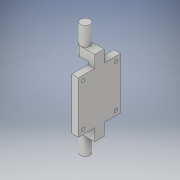
# Autodesk Inventor part: Paltte klein 2.0
Saved by Autodesk Inventor 2018.3 (Build 223284000, 284)
## iProperties
Created: 2018-11-08
Part Number: Paltte klein 2.0
Material: Generisch
Document SubType Name: Modeling
Designer: pgmadmin
Density: 1 g/cm^3
Appearance: Vorgabe
Author: pgmadmin
Autodesk Inventor part; units mm, degrees
ref_plane "YZ Plane" through (0, 0, 0) normal (1, 0, 0) x (0, 1, 0)
ref_plane "XZ Plane" through (0, 0, 0) normal (0, 1, 0) x (-1, 0, 0)
ref_plane "XY Plane" through (0, 0, 0) normal (0, 0, 1) x (1, 0, 0)
sketch "Skizze1" plane through (0, 0, 0) normal (1, 0, 0) x (0, 1, 0)
  line L0 (52.9121, 68.8462) -> (7.9121, 68.8462)
  line L1 (7.9121, 68.8462) -> (7.9121, 13.8462)
  line L2 (7.9121, 13.8462) -> (52.9121, 13.8462)
  line L3 (52.9121, 13.8462) -> (52.9121, 68.8462)
  circle A0 centre (12.9121, 18.8462) radius 1.75
  circle A1 centre (12.9121, 63.8462) radius 1.75
  circle A2 centre (47.9121, 63.8462) radius 1.75
  circle A3 centre (47.9121, 18.8462) radius 1.75
  point P0 (0, 0)
  dimension "d0" = 45
  dimension "d1" = 55
  dimension "d2" = 3.5
  dimension "d3" = 5
  dimension "d4" = 5
  dimension "d5" = 3.5
  dimension "d6" = 5
  dimension "d7" = 3.5
  dimension "d8" = 5
  dimension "d11" = 3.5
  constraints: 8 end point, 4 centre point, 4 coincident, 2 parallel, 1 horizontal, 1 perpendicular
  measures "d0" distance of L1.end L2.end
  measures "d1" distance of L0.end L1.end
  measures "d2" diameter of A0
  measures "d3" distance from line of L1 A0.centre
  measures "d4" distance from line of L2 A0.centre
  measures "d5" diameter of A1
  measures "d6" distance from line of L0 A1.centre
  measures "d7" diameter of A2
  measures "d8" distance from line of L3 A2.centre
  measures "d11" diameter of A3
extrude "Extrusion1" add sketch "Skizze1" along normal blind 7
sketch "Skizze2" plane through (0, 7.9121, 68.8462) normal (0, 0, 1) x (1, 0, 0)
  line L0 (0, 45) -> (0, 0) projected
  line L1 (7, 45) -> (7, 0) projected
  line L2 (0, 17.5) -> (7, 17.5)
  line L3 (7, 17.5) -> (7, 27.5)
  line L4 (7, 27.5) -> (0, 27.5)
  line L5 (0, 27.5) -> (0, 17.5)
  line L6 (0, 45) -> (7, 45) projected
  point P0 (0, -7.9121)
  dimension "d12" = 17.5
  dimension "d13" = 10
  constraints: 8 end point, 2 parallel, 2 point on line, 1 horizontal, 1 perpendicular
  measures "d12" distance between parallel lines of L6 L4
  measures "d13" distance between parallel lines of L4 L2
extrude "Extrusion2" add sketch "Skizze2" along normal blind 13 contours L4 L1 L2 L0
sketch "Skizze3" plane through (0, 7.9121, 13.8462) normal (0, 0, -1) x (-1, 0, 0)
  line L0 (0, 0) -> (0, 45) projected
  line L1 (-7, 27.5) -> (0, 27.5)
  line L2 (0, 27.5) -> (0, 17.5)
  line L3 (0, 17.5) -> (-7, 17.5)
  line L4 (-7, 17.5) -> (-7, 27.5)
  line L5 (0, 0) -> (-7, 0) projected
  point P0 (0, -7.9121)
  dimension "d16" = 10
  dimension "d17" = 17.5
  dimension "d18" = 7
  constraints: 8 end point, 2 parallel, 1 horizontal, 1 perpendicular, 1 point on line
  measures "d16" distance between parallel lines of L3 L1
  measures "d17" distance between parallel lines of L5 L3
  measures "d18" distance between parallel lines of L0 L4
extrude "Extrusion3" add sketch "Skizze3" along normal blind 13
sketch "Skizze4" plane through (0, 0, 0) normal (-1, 0, 0) x (0, 0, 1)
  line L0 (13.8462, 25.4121) -> (0.8462, 25.4121) projected
  line L1 (13.8462, 35.4121) -> (0.8462, 35.4121) projected
  line L2 (0.8462, 25.4121) -> (10.8462, 25.4121)
  line L3 (10.8462, 25.4121) -> (10.8462, 35.4121)
  line L4 (10.8462, 35.4121) -> (0.8462, 35.4121)
  line L5 (0.8462, 35.4121) -> (0.8462, 25.4121)
  line L6 (81.8462, 25.4121) -> (81.8462, 35.4121) projected
  line L7 (68.8462, 35.4121) -> (81.8462, 35.4121) projected
  line L8 (81.8462, 25.4121) -> (71.8462, 25.4121)
  line L9 (71.8462, 25.4121) -> (71.8462, 35.4121)
  line L10 (71.8462, 35.4121) -> (81.8462, 35.4121)
  line L11 (81.8462, 35.4121) -> (81.8462, 25.4121)
  point P0 (0, 0)
  dimension "d21" = 10
  dimension "d22" = 10
  constraints: 16 end point, 4 parallel, 2 horizontal, 2 perpendicular, 2 point on line
  measures "d21" distance of L4.end L3.end
  measures "d22" distance of L9.end L10.end
extrude "Extrusion4" add sketch "Skizze4" along normal blind 12
sketch "Skizze5" plane through (0, 7.9121, 81.8462) normal (0, 0, 1) x (1, 0, 0)
  circle A0 centre (-8, 22.5) radius 5
  line L0 (7, 17.5) -> (-12, 17.5) projected
  line L1 (-12, 17.5) -> (-12, 27.5) projected
  point P0 (0, -7.9121)
  dimension "d25" = 10
  dimension "d26" = 5
  dimension "d27" = 4
  constraints: 1 centre point
  measures "d25" diameter of A0
  measures "d26" distance from line of L0 A0.centre
  measures "d27" distance from line of A0.centre L1
extrude "Extrusion5" add sketch "Skizze5" along normal blind 20 contours A0 L1 | L1 A0
sketch "Skizze6" plane through (0, 7.9121, 0.8462) normal (0, 0, -1) x (-1, 0, 0)
  circle A0 centre (8, 22.5) radius 5
  line L0 (12, 27.5) -> (12, 17.5) projected
  line L1 (-7, 17.5) -> (12, 17.5) projected
  point P0 (0, -7.9121)
  dimension "d30" = 10
  dimension "d31" = 4
  dimension "d47" = 5
  constraints: 1 centre point
  measures "d30" diameter of A0
  measures "d31" distance from line of A0.centre L0
  measures "d47" distance from line of L1 A0.centre
extrude "Extrusion6" add sketch "Skizze6" along normal blind 20 contours A0 L0 | L0 A0
fillet "Rundung1" radius 4 1 edges at (-12, 35.4121, 76.8462)
fillet "Rundung2" radius 3 3 edges at (-12, 25.4121, 76.8462) (-12, 25.4121, 5.8462) (-12, 35.4121, 5.8462)
sketch "Skizze7" plane through (0, 0, 0) normal (-1, 0, 0) x (0, 0, 1)
  circle A0 centre (18.8462, 47.9121) radius 1.75 projected
  circle A1 centre (18.8462, 12.9121) radius 1.75 projected
  circle A2 centre (63.8462, 12.9121) radius 1.75 projected
  point P0 (0, 0)
  point P1 (63.8462, 47.9121)
  dimension "d36" = 0
  dimension "d37" = 0
  dimension "d38" = 0
  dimension "d39" = 0
  measures "d36" distance of A0.centre point (18.846, 47.912)
  measures "d37" distance of A0.centre point (18.846, 47.912)
  measures "d38" distance of A1.centre point (18.846, 12.912)
  measures "d39" distance of A2.centre point (63.846, 12.912)
hole "Bohrung1" at (0, 47.9121, 18.8462) at (0, 12.9121, 18.8462) at (0, 12.9121, 63.8462) at (0, 47.9121, 63.8462) direction (1, 0, 0) diameter 6.5 depth 2.25 tip angle 118
